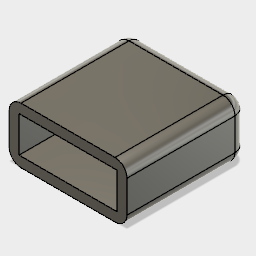
USB_Cap (Autodesk Fusion 360 design; units mm, degrees)
Autodesk Fusion 360 part; units mm, degrees
sketch "Sketch1" plane through (0, 0, 0) normal (0, 1, 0) x (1, 0, 0)
  line L0 (-7.375, 7.5) -> (7.375, 7.5)
  line L1 (7.375, 7.5) -> (7.375, -7.5)
  line L2 (7.375, -7.5) -> (-7.375, -7.5)
  line L3 (-7.375, -7.5) -> (-7.375, 7.5)
  line L4 (-7.375, 7.5) -> (7.375, -7.5) construction
  line L5 (7.375, 7.5) -> (-7.375, -7.5) construction
  line L6 (-6.125, 6.25) -> (6.125, 6.25)
  line L7 (6.125, 6.25) -> (6.125, -6.25)
  line L8 (6.125, -6.25) -> (-6.125, -6.25)
  line L9 (-6.125, -6.25) -> (-6.125, 6.25)
  line L10 (-6.125, 6.25) -> (6.125, -6.25) construction
  line L11 (6.125, 6.25) -> (-6.125, -6.25) construction
  line L12 (-6.125, -6.25) -> (-6.125, -7.5)
  line L13 (6.125, -6.25) -> (6.125, -7.5)
  dimension "d1" = 15
  dimension "d2" = 14.75
  dimension "d5" = 12.25
  dimension "d6" = 12.5
  constraint perpendicular L0 L1
  constraint parallel L0 L2
  constraint parallel L1 L3
  constraint horizontal L0
  constraint coincident L4 origin
  constraint coincident L5 origin
  constraint perpendicular L6 L7
  constraint parallel L6 L8
  constraint parallel L7 L9
  constraint horizontal L6
  constraint coincident L10 origin
  constraint coincident L11 origin
  constraint coincident L2 origin
  constraint perpendicular L2 L12
  constraint coincident L2
  constraint perpendicular L2 L13
  measures "d1" distance of origin
  measures "d2" distance of origin
extrude "Extrude1" add sketch "Sketch1" along normal blind 1.25 makes body 1
extrude "Extrude2" add sketch "Sketch1" along normal blind 5.75 contours L0 L1 L2 L3 L6 L7 L9 L12 L13 bodies 1
extrude "Extrude3" add sketch "Sketch1" along normal blind 1.25 separate body makes body 2
move_body "MoveBody1" bodies 2 to x (1, 0, 0) y (0, 1, 0) z (0, 0, 1) at (0, 5.75, 0)
combine "Combine1" operation add target body 1 tool bodies 2
fillet "Fillet1" radius 1.5 8 edges at (-7.375, 7, 0) (-7.375, 0, 0) (0, 0, -7.5) (7.375, 0, 0) (7.375, 7, 0) (0, 7, -7.5) (-7.375, 3.5, -7.5) (7.375, 3.5, -7.5) on bodies 1
